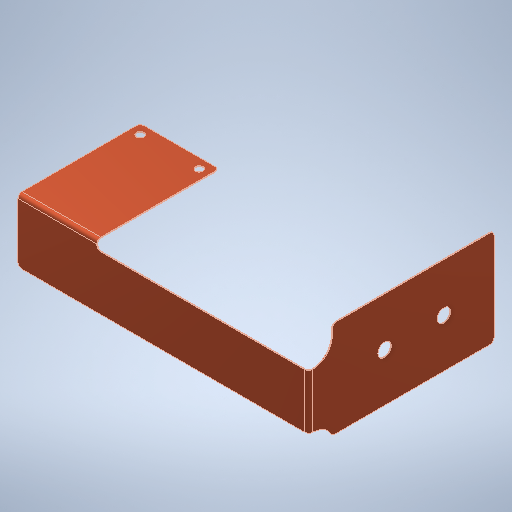
# Autodesk Inventor part: Flex V1
Saved by Autodesk Inventor 2025 (Build 290162000, 162)
## iProperties
Created: 2024-08-07
Part Number: Flex V1
Material: Copper
Document SubType Name: Modeling
Designer: Caleb Fangmeier
Density: 8.94 g/cm^3
Appearance: Copper - Satin
Author: Caleb Fangmeier
Autodesk Inventor part; units mm, degrees
ref_plane "YZ Plane" through (0, 0, 0) normal (1, 0, 0) x (0, 1, 0)
ref_plane "XZ Plane" through (0, 0, 0) normal (0, 1, 0) x (-1, 0, 0)
ref_plane "XY Plane" through (0, 0, 0) normal (0, 0, 1) x (1, 0, 0)
sketch "Sketch1" plane through (0, 0, 0) normal (0, 1, 0) x (-1, 0, 0)
  line L0 (-10, -11.1404) -> (10, -11.1404)
  line L1 (10, -11.1404) -> (10, 18.8596)
  line L2 (10, 18.8596) -> (-10, 18.8596)
  line L3 (-10, 18.8596) -> (-10, -11.1404)
  point P0 (0, 0)
  dimension "d0" = 20
  dimension "d1" = 10
  dimension "d2" = 30
  constraints: 8 end point, 2 parallel, 1 horizontal, 1 perpendicular
  measures "d0" distance of L0.start L0.end
  measures "d1" distance from line of L1 point (0, 0)
  measures "d2" distance of L0.end L1.end
extrude "Extrusion1" add sketch "Sketch1" along normal blind 0.2
sketch "Sketch2" plane through (10, 0, 18.8596) normal (1, 0, 0) x (0, 0, -1)
  line L0 (30, 0.2) -> (0, 0.2) projected
  arc A0 (0, 0.2) -> (-1, -0.8) centre (0, -0.8) ccw
  line L1 (0, -0.8) -> (-1, -0.8) construction
  line L2 (0, -0.8) -> (0, 0.2) construction
  arc A1 (0, 0) -> (-0.8, -0.8) centre (0, -0.8) ccw
  line L3 (0, 0) -> (30, 0) projected
  line L4 (-0.8, -0.8) -> (-0.8, -15.8)
  line L5 (-0.8, -15.8) -> (-1, -15.8)
  line L6 (-1, -15.8) -> (-1, -0.8)
  line L7 (0, 0) -> (0, 0.2) projected
  point P0 (18.8596, 0)
  dimension "d5" = 90
  dimension "d6" = 1
  dimension "d7" = 0.2
  dimension "d8" = 0.2
  dimension "d9" = 15
  constraints: 10 end point, 4 point on circle, 2 centre point, 2 point on line, 1 coincident, 1 parallel, 1 vertical alignment
  measures "d5" angle of L2 L1
  measures "d6" radius of A0
  measures "d7" distance between parallel lines of L0 L3
  measures "d8" radial gap between concentric circles of A0 A1
  measures "d9" distance of L5.end L1.end
extrude "Extrusion2" add sketch "Sketch2" against normal up to surface (20 mm away)
sketch "Sketch3" plane through (10, -15.8, 19.8596) normal (1, 0, 0) x (0, 0, -1)
  arc A0 (1, 16) -> (0, 15) centre (1, 15) ccw projected
  arc A1 (1, 15.8) -> (0.2, 15) centre (1, 15) ccw projected
  line L0 (0, 13.8) -> (0.2, 13.8)
  line L1 (0, 15) -> (0, 0) projected
  line L2 (0.2, 0) -> (0.2, 15) projected
  line L3 (0, 0) -> (0.2, 0) projected
  point P0 (19.8596, 15.8)
  dimension "d19" = 1.2
  constraints: 2 end point, 2 point on line, 1 horizontal
  measures "d19" distance from line of L0 L2.end
extrude "Extrusion3" add sketch "Sketch3" along normal blind 52.7
sketch "Sketch4" plane through (10, -2, 19.8596) normal (0, 1, 0) x (1, 0, 0)
  line L0 (52.7, 0.2) -> (52.7, 0) projected
  arc A0 (52.7, 0) -> (53.7, 1) centre (52.7, 1) ccw
  line L1 (52.7, 1) -> (53.7, 1) construction
  line L2 (52.7, 1) -> (52.7, 0) construction
  arc A1 (52.7, 0.2) -> (53.5, 1) centre (52.7, 1) ccw
  line L3 (53.5, 1) -> (53.5, 47)
  line L4 (53.5, 47) -> (53.7, 47)
  line L5 (53.7, 47) -> (53.7, 1)
  point P0 (-10, 19.8596)
  dimension "d14" = 90
  dimension "d15" = 1
  dimension "d16" = 46
  dimension "d28" = 0.2
  constraints: 10 end point, 4 point on circle, 2 centre point, 2 vertical alignment, 1 coincident, 1 horizontal alignment, 1 parallel, 1 point on line, 1 tangent
  measures "d14" angle of L2 L1
  measures "d15" radius of A0
  measures "d16" distance of L4.end L1.end
  measures "d28" distance of L0.start L2.end
extrude "Extrusion4" add sketch "Sketch4" against normal up to surface (13.8 mm away)
sketch "Sketch5" plane through (63.7, -2, 18.8596) normal (1, 0, 0) x (0, 0, -1)
  line L0 (46, 0) -> (0, 0) projected
  line L1 (0, 0) -> (0, 0)
  line L2 (46, 0) -> (46, 7.5)
  line L3 (46, 7.5) -> (5, 7.5)
  line L4 (5, 7.5) -> (5, 5)
  arc A0 (0, 0) -> (5, 5) centre (0, 5) ccw
  point P0 (18.8596, 2)
  point P1 (5, 6.25)
  point P2 (30, 0)
  dimension "d20" = 7.5
  dimension "d21" = 5
  dimension "d22" = 5
  constraints: 8 end point, 2 parallel, 2 point on circle, 2 tangent, 1 centre point, 1 horizontal, 1 midpoint, 1 perpendicular, 1 point on line
  measures "d20" distance of L0.start L2.end
  measures "d21" horizontal distance of point (5, 6.25) L0.end
  measures "d22" radius of A0
extrude "Extrusion5" add sketch "Sketch5" against normal up to surface (0.2 mm away)
sketch "Sketch6" plane through (63.7, -15.8, 18.8596) normal (1, 0, 0) x (0, 0, -1)
  line L0 (46, 0) -> (46, 21.3) projected
  line L1 (46, 0) -> (5, 0)
  line L2 (5, -3.2119) -> (46, -3.2119)
  line L3 (46, -3.2119) -> (46, 0)
  line L4 (5, 21.3) -> (5, 18.8) projected
  line L5 (46, 0) -> (0, 0) projected
  arc A0 (5, -3.2119) -> (0, 0) centre (0, -5.4977) ccw
  line L6 (-1, 0) -> (0, 0) projected
  line L7 (0, 0) -> (5, 0)
  point P0 (18.8596, 15.8)
  point P1 (46.1737, 13.8)
  constraints: 8 end point, 2 point on circle, 2 tangent, 1 centre point, 1 collinear, 1 horizontal, 1 parallel, 1 vertical alignment, 1 other
extrude "Extrusion6" add sketch "Sketch6" against normal up to surface (0.2 mm away)
fillet "Fillet1" radius 1 8 edges at (63.6, 5.5, 13.8596) (63.6, 5.5, -27.1404) (63.6, -19.0119, -27.1404) (63.6, -19.0119, 13.8596) (10, 0.1, -11.1404) (-10, 0.1, -11.1404) (-10, -15.8, 19.7596) (10, -2, 19.7596)
sketch "Sketch7" plane through (0, 0.2, 0) normal (0, 1, 0) x (1, 0, 0)
  line L0 (-10, 10.1404) -> (-10, -18.8596) projected
  line L1 (9, 11.1404) -> (-9, 11.1404) projected
  line L2 (10, -18.8596) -> (10, 10.1404) projected
  point P0 (0, 0)
  point P1 (7.5, 8.6404)
  point P2 (-7.5, 8.6404)
  dimension "d29" = 2.5
  dimension "d30" = 2.5
  dimension "d31" = 2.5
  constraints: 1 horizontal alignment
  measures "d29" distance from line of L0 point (-7.5, 8.64)
  measures "d30" distance from line of L1 point (-7.5, 8.64)
  measures "d31" distance from line of L2 point (7.5, 8.64)
hole "Hole1" at (7.5, 0.2, -8.6404) at (-7.5, 0.2, -8.6404) direction (0, -1, 0) diameter 2 depth 7.9 tip angle 118
sketch "Sketch8" plane through (63.7, -15.8, 18.8596) normal (1, 0, 0) x (0, 0, -1)
  line L0 (45, 21.3) -> (6, 21.3) projected
  line L1 (5.6057, -3.2119) -> (45, -3.2119) projected
  line L2 (46, -2.2119) -> (46, 20.3) projected
  point P0 (18.8596, 15.8)
  point P1 (18.26, 9.044)
  point P2 (33.26, 9.044)
  dimension "d39" = 24.5119
  dimension "d40" = 12.256
  dimension "d41" = 15
  dimension "d42" = 12.74
  constraints: 1 horizontal alignment
  measures "d39" distance between parallel lines of L0 L1
  measures "d40" distance from line of L1 point (18.26, 9.044)
  measures "d41" distance of point (33.26, 9.044) point (18.26, 9.044)
  measures "d42" distance from line of L2 point (33.26, 9.044)
hole "Hole2" at (63.7, -6.756, 0.5996) at (63.7, -6.756, -14.4004) direction (-1, 0, 0) diameter 3.4 depth 7.9 tip angle 118 clearance for "Flat Head Machine Screw" size "M3" standard "Ansi Metric M Profile"
equation "\"d1\" = 0.5 * d0"
equation "\"d8\" = d7"
equation "\"d30\" = d29"
equation "\"d31\" = d29"
equation "\"d40\" = 0.5 * d39"
body "Solid1"
